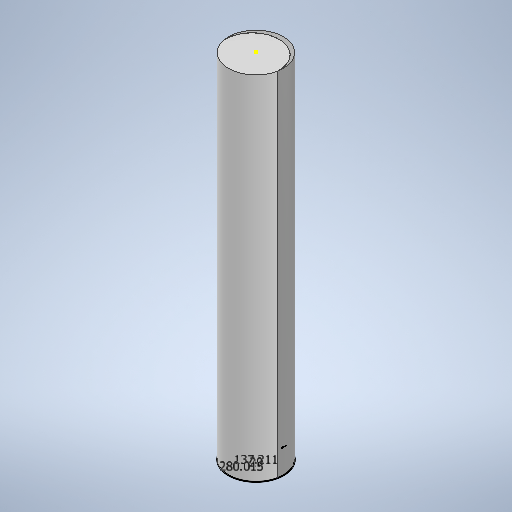
# Autodesk Inventor part: control drum
Saved by Autodesk Inventor 2025.2 (Build 292293000, 293)
## iProperties
Created: 2025-04-27
Part Number: control drum
Material: Generic
Document SubType Name: Modeling
Designer: alex
Density: 1 g/cm^3
Appearance: Default
Author: alex
Autodesk Inventor part; units mm, degrees
ref_plane "YZ Plane" through (0, 0, 0) normal (1, 0, 0) x (0, 1, 0)
ref_plane "XZ Plane" through (0, 0, 0) normal (0, 1, 0) x (-1, 0, 0)
ref_plane "XY Plane" through (0, 0, 0) normal (0, 0, 1) x (1, 0, 0)
sketch "Sketch1" plane through (0, 0, 0) normal (0, 1, 0) x (-1, 0, 0)
  circle A0 centre (0, 0) radius 140.0075
  arc A1 (-136.8898, 29.3816) -> (136.8898, 29.3816) centre (0, 20) ccw
  dimension "d0" = 280.015
  dimension "d1" = 20
  dimension "d4" = 137.2109
  constraints: 4 point on circle, 2 centre point, 1 coincident
  measures "d0" diameter of A0
  measures "d1" distance of point (0, 0) A1.centre
  measures "d4" radius of A1
extrude "Extrusion1" add sketch "Sketch1" along normal blind 1800 contours A1 A0 picked at (0, 54.1051)
sketch "Sketch2" plane through (0, 1800, 0) normal (0, 1, 0) x (1, 0, 0)
  point P0 (0, 0)
extrude "Extrusion2" add sketch "Sketch1" along normal blind 1800 separate body contours A0 A1 picked at (8.5009, -124.3896)
body "Solid1"
body "Solid2"
